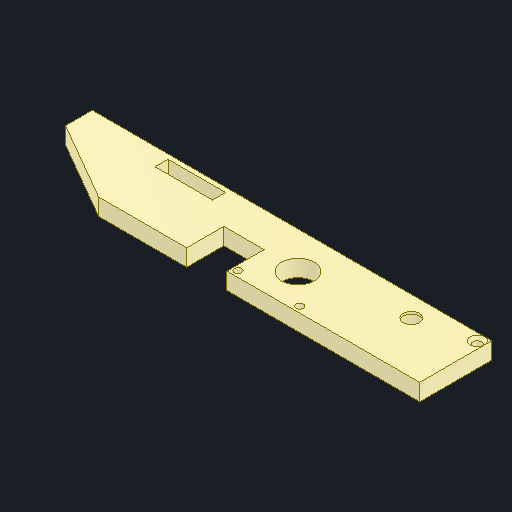
# Autodesk Inventor part: right_hold
Saved by Autodesk Inventor 2023 (Build 270158000, 158)
## iProperties
Created: 2024-04-29
Part Number: right_hold
Material: Nylon 6/6
Document SubType Name: Modeling
Designer: szymo
Density: 1.13 g/cm^3
Appearance: Nylon 6
Mass: 31.6817 g
Surface Area: 122.994 cm^2
Volume: 28.0369 cm^3
Author: szymo
Autodesk Inventor part; units mm, degrees
(part 1 of 2)
ref_plane "YZ Plane" through (0, 0, 0) normal (1, 0, 0) x (0, 1, 0)
ref_plane "XZ Plane" through (0, 0, 0) normal (0, 1, 0) x (-1, 0, 0)
ref_plane "XY Plane" through (0, 0, 0) normal (0, 0, 1) x (1, 0, 0)
sketch "Sketch1" plane through (0, 0, 0) normal (0, 0, 1) x (1, 0, 0)
  line L0 (91, -34) -> (91, 34) projected
  line L1 (91, 34) -> (41, 34) projected
  line L2 (41, 34) -> (41, 89) projected
  line L3 (41, 89) -> (-91, 89) projected
  line L4 (-91, 89) -> (-91, -89) projected
  line L5 (-91, -89) -> (41, -89) projected
  line L6 (41, -89) -> (41, -34) projected
  line L7 (41, -34) -> (91, -34) projected
  line L8 (70, 27) -> (62, 27) projected
  line L9 (91, 34) -> (-87, 34)
  line L10 (-87, 34) -> (-87, 27)
  line L11 (-87, 27) -> (91, 27)
  line L12 (91, 27) -> (91, 34)
  circle A0 centre (-83, 21.5) radius 1.2295 projected
  circle A1 centre (-83, -64.5) radius 1.2295 projected
  circle A2 centre (-83, -21.5) radius 1.2295 projected
  circle A3 centre (-83, 64.5) radius 1.2295 projected
  line L13 (-85, -72) -> (-76, -72) projected
  line L14 (-76, -72) -> (-76, -57) projected
  line L15 (-76, -57) -> (-85, -57) projected
  arc A4 (-87, -55) -> (-85, -57) centre (-85, -55) ccw projected
  line L16 (-87, -55) -> (-87, -31) projected
  arc A5 (-85, -29) -> (-87, -31) centre (-85, -31) ccw projected
  line L17 (-85, -29) -> (-76, -29) projected
  line L18 (-76, -29) -> (-76, -14) projected
  line L19 (-76, -14) -> (-85, -14) projected
  arc A6 (-87, -12) -> (-85, -14) centre (-85, -12) ccw projected
  line L20 (-87, -12) -> (-87, 12) projected
  arc A7 (-85, 14) -> (-87, 12) centre (-85, 12) ccw projected
  line L21 (-85, 14) -> (-76, 14) projected
  line L22 (-76, 14) -> (-76, 29) projected
  line L23 (-76, 29) -> (-85, 29) projected
  arc A8 (-87, 31) -> (-85, 29) centre (-85, 31) ccw projected
  line L24 (-87, 31) -> (-87, 55) projected
  arc A9 (-85, 57) -> (-87, 55) centre (-85, 55) ccw projected
  line L25 (-85, 57) -> (-76, 57) projected
  line L26 (-76, 57) -> (-76, 72) projected
  line L27 (-76, 72) -> (-85, 72) projected
  arc A10 (-87, 74) -> (-85, 72) centre (-85, 74) ccw projected
  line L28 (-87, 74) -> (-87, 89) projected
  line L29 (-91, 89) -> (-87, 89) projected
  line L30 (-91, -89) -> (-91, 89) projected
  line L31 (-91, -89) -> (-87, -89) projected
  line L32 (-87, -89) -> (-87, -74) projected
  arc A11 (-85, -72) -> (-87, -74) centre (-85, -74) ccw projected
  line L33 (-91, 89.5) -> (-86.5, 89.5)
  line L34 (-86.5, 89.5) -> (-86.5, 74)
  arc A12 (-86.5, 74) -> (-85, 72.5) centre (-85, 74) ccw
  line L35 (-85, 72.5) -> (-75.5, 72.5)
  line L36 (-75.5, 72.5) -> (-75.5, 56.5)
  line L37 (-75.5, 56.5) -> (-85, 56.5)
  arc A13 (-85, 56.5) -> (-86.5, 55) centre (-85, 55) ccw
  line L38 (-86.5, 55) -> (-86.5, 31)
  arc A14 (-86.5, 31) -> (-85, 29.5) centre (-85, 31) ccw
  line L39 (-85, 29.5) -> (-75.5, 29.5)
  line L40 (-75.5, 29.5) -> (-75.5, 13.5)
  line L41 (-75.5, 13.5) -> (-85, 13.5)
  arc A15 (-85, 13.5) -> (-86.5, 12) centre (-85, 12) ccw
  line L42 (-86.5, 12) -> (-86.5, -12)
  arc A16 (-86.5, -12) -> (-85, -13.5) centre (-85, -12) ccw
  line L43 (-85, -13.5) -> (-75.5, -13.5)
  line L44 (-75.5, -13.5) -> (-75.5, -29.5)
  line L45 (-75.5, -29.5) -> (-85, -29.5)
  arc A17 (-85, -29.5) -> (-86.5, -31) centre (-85, -31) ccw
  line L46 (-86.5, -31) -> (-86.5, -55)
  arc A18 (-86.5, -55) -> (-85, -56.5) centre (-85, -55) ccw
  line L47 (-85, -56.5) -> (-75.5, -56.5)
  line L48 (-75.5, -56.5) -> (-75.5, -72.5)
  line L49 (-75.5, -72.5) -> (-85, -72.5)
  arc A19 (-85, -72.5) -> (-86.5, -74) centre (-85, -74) ccw
  line L50 (-86.5, -74) -> (-86.5, -89.5)
  line L51 (-86.5, -89.5) -> (-91, -89.5)
  line L52 (-86.5, 31) -> (-75.5, 31)
  line L53 (-75.5, 31) -> (-75.5, 29.5)
  line L54 (-75.5, 31) -> (-75.5, 34)
  point P0 (0, 0)
  point P1 (-75.5, 27)
  point P2 (-86.5, 34)
  dimension "d6" = 0.5
  constraints: 52 end point, 16 point on circle, 8 centre point, 3 perpendicular, 2 collinear, 2 horizontal, 2 parallel, 1 point on line, 26 other
  measures "d6" distance between parallel lines of L22 L40
extrude "Extrusion1" add sketch "Sketch1" along normal blind 30 contours L11 L8 L40 L53 L54 L9 L1 L0
sketch "Sketch3" plane through (-86.5, 34, 0) normal (0, 1, 0) x (1, 0, 0)
  line L0 (-0.5, -4.5) -> (-0.5, 0) projected
  line L1 (-0.5, 0) -> (-4.5, 0) projected
  line L2 (-4.5, 0) -> (-4.5, 3.5) projected
  line L3 (-4.5, 3.5) -> (-18.5, 3.5) projected
  line L4 (-18.5, 3.5) -> (-4.5, -5.5) projected
  line L5 (-4.5, -5.5) -> (-4.5, -4.5) projected
  line L6 (-4.5, -4.5) -> (-0.5, -4.5) projected
  line L7 (-0.5, -4.5) -> (50.0525, -33.6865)
  line L8 (177.5, 0) -> (11, 0) projected
  line L9 (177.5, -30) -> (11, -30) projected
  line L10 (177.5, 0) -> (177.5, -30) projected
  line L11 (11, 0) -> (11, -30) projected
  point P0 (86.5, 0)
  point P1 (43.6673, -30)
  point P2 (11, -11.1395)
  dimension "d7" = 30
  constraints: 2 end point
  measures "d7" angle of L7 L6
extrude "Extrusion4" cut sketch "Sketch3" against normal blind 30 contours L7 L9 L11
sketch "Sketch5" plane through (-75.5, 27, 0) normal (0, -1, 0) x (1, 0, 0)
  line L0 (56.5, 7.0341) -> (57.5, 7.0341) projected
  line L1 (34.5, 7.0341) -> (56.5, 7.0341) projected
  line L2 (33.5, 7.0341) -> (33.5, 6.6226)
  line L3 (33.5, 6.6226) -> (9.5, 6.6226)
  line L4 (9.5, 6.6226) -> (9.5, 7.0341)
  line L5 (9.5, 7.0341) -> (33.5, 7.0341)
  line L6 (64.5, 7.0341) -> (64.5, 6.6226)
  line L7 (64.5, 6.6226) -> (57.5, 6.6226)
  line L8 (57.5, 6.6226) -> (57.5, 7.0341)
  line L9 (57.5, 7.0341) -> (64.5, 7.0341)
  line L10 (9.5, 2) -> (9.5, 2.6226)
  line L11 (9.5, 2.6226) -> (64.5, 2.6226)
  line L12 (64.5, 2.6226) -> (64.5, 2)
  line L13 (64.5, 2) -> (9.5, 2)
  line L14 (9.5, 7.0341) -> (64.5, 7.0341)
  line L15 (64.5, 7.0341) -> (64.5, 2)
  line L16 (64.5, 2) -> (9.5, 2)
  line L17 (9.5, 2) -> (9.5, 7.0341)
  line L18 (9.2, 7.3341) -> (64.8, 7.3341)
  line L19 (64.8, 7.3341) -> (64.8, 1.9)
  line L20 (64.8, 1.9) -> (9.2, 1.9)
  line L21 (9.2, 1.9) -> (9.2, 7.3341)
  point P0 (75.5, 0)
  dimension "d19" = 0.3
  dimension "d20" = 0.3
  dimension "d21" = 0.1
  dimension "d22" = 0.3
  constraints: 40 end point, 8 horizontal, 6 vertical, 4 parallel, 2 perpendicular, 11 other
  measures "d19" distance between parallel lines of L21 L17
  measures "d20" distance between parallel lines of L19 L15
  measures "d21" distance between parallel lines of L13 L20
  measures "d22" distance between parallel lines of L18 L1
extrude "Extrusion6" cut sketch "Sketch5" against normal blind 0.7 contours L0 L8 L7 L15 L11 L17 L3 L2 L14 L1 | L9 L6 L7 L8 | L2 L3 L4 L5 | L12 L13 L10 L11 | L18 L19 L20 L21
sketch "Sketch6" plane through (-75.5, 27, 0) normal (0, -1, 0) x (1, 0, 0)
  line L0 (33.5, 7.0341) -> (34.5, 7.0341) projected
  line L1 (34.5, 7.0341) -> (56.5, 7.0341) projected
  line L2 (56.5, 7.0341) -> (57.5, 7.0341) projected
  line L3 (64.8, 1.9) -> (9.2, 1.9) projected
  line L4 (64.8, 7.3341) -> (64.8, 1.9) projected
  line L5 (9.2, 7.3341) -> (64.8, 7.3341) projected
  line L6 (9.2, 1.9) -> (9.2, 7.3341) projected
  line L7 (33.5, 7.3341) -> (57.5, 7.3341)
  line L8 (57.5, 7.3341) -> (57.5, 1.9)
  line L9 (57.5, 1.9) -> (33.5, 1.9)
  line L10 (33.5, 1.9) -> (33.5, 7.3341)
  point P0 (75.5, 0)
  constraints: 8 end point, 4 point on line, 2 parallel, 1 horizontal, 1 perpendicular
extrude "Extrusion7" cut sketch "Sketch6" against normal up to next contours L10 L5 L8 L2 L1 L0 | L0 L1 L2 L8 L3 L10
sketch "Sketch7" plane through (0, 0, 30) normal (0, 0, 1) x (1, 0, 0)
  line L0 (10.25, -34) -> (10.25, 34) projected
  line L1 (10.25, 34) -> (-5.75, 34) projected
  line L2 (-5.75, -34) -> (-5.75, 34) projected
  line L3 (10.25, -34) -> (-5.75, -34) projected
  line L4 (-42.8327, 27) -> (91, 27) projected
  line L5 (10.25, 34) -> (-5.75, 34)
  line L6 (-5.75, 34) -> (-5.75, 27)
  line L7 (-5.75, 27) -> (10.25, 27)
  line L8 (10.25, 27) -> (10.25, 34)
  line L9 (10.65, 34) -> (-6.15, 34)
  line L10 (-6.15, 34) -> (-6.15, 27)
  line L11 (-6.15, 27) -> (10.65, 27)
  line L12 (10.65, 27) -> (10.65, 34)
  point P0 (0, 0)
  dimension "d27" = 0.4
  dimension "d28" = 0.4
  constraints: 16 end point, 4 parallel, 4 point on line, 2 horizontal, 2 perpendicular
  measures "d27" distance between parallel lines of L12 L0
  measures "d28" distance between parallel lines of L2 L10
extrude "Extrusion8" cut sketch "Sketch7" against normal blind 15.5 contours L4 L2 L1 L0 | L0 L9 L12 L4 | L4 L10 L9 L2
sketch "Sketch9" plane through (91, 27, 0) normal (0, -1, 0) x (1, 0, 0)
  arc A0 (-67.8175, 18.3693) -> (-69.7313, 19.2694) centre (-70.7618, 14.5935) ccw projected
  arc A1 (-69.7313, 19.2694) -> (-70.2869, 18.54) centre (-65.375, 15.375) ccw projected
  arc A2 (-70.2869, 18.54) -> (-68.9106, 16.9341) centre (-66.053, 20.7758) ccw projected
  arc A3 (-68.9106, 16.9341) -> (-69.111, 16.3618) centre (-65.375, 15.375) ccw projected
  arc A4 (-69.111, 16.3618) -> (-71.1884, 15.965) centre (-69.2737, 11.5765) ccw projected
  arc A5 (-71.1884, 15.965) -> (-71.2091, 15.0484) centre (-65.375, 15.375) ccw projected
  arc A6 (-71.2091, 15.0484) -> (-69.1518, 14.5581) centre (-69.098, 19.3459) ccw projected
  arc A7 (-69.1518, 14.5581) -> (-68.9775, 13.9774) centre (-65.375, 15.375) ccw projected
  arc A8 (-68.9775, 13.9774) -> (-70.425, 12.4353) centre (-66.2964, 10.0103) ccw projected
  arc A9 (-70.425, 12.4353) -> (-69.9029, 11.6815) centre (-65.375, 15.375) ccw projected
  arc A10 (-69.9029, 11.6815) -> (-67.9503, 12.4942) centre (-70.721, 16.3992) ccw projected
  arc A11 (-67.9503, 12.4942) -> (-67.468, 12.1268) centre (-65.375, 15.375) ccw projected
  arc A12 (-67.468, 12.1268) -> (-67.7326, 10.0285) centre (-62.9672, 10.4933) ccw projected
  arc A13 (-67.7326, 10.0285) -> (-66.8672, 9.7255) centre (-65.375, 15.375) ccw projected
  arc A14 (-66.8672, 9.7255) -> (-65.7652, 11.5306) centre (-70.302, 13.0613) ccw projected
  arc A15 (-65.7652, 11.5306) -> (-65.159, 11.5169) centre (-65.375, 15.375) ccw projected
  arc A16 (-65.159, 11.5169) -> (-64.1397, 9.6638) centre (-60.5576, 12.8409) ccw projected
  arc A17 (-64.1397, 9.6638) -> (-63.2615, 9.9273) centre (-65.375, 15.375) ccw projected
  arc A18 (-63.2615, 9.9273) -> (-63.431, 12.0355) centre (-68.0011, 10.6071) ccw projected
  arc A19 (-63.431, 12.0355) -> (-62.9325, 12.3807) centre (-65.375, 15.375) ccw projected
  arc A20 (-62.9325, 12.3807) -> (-61.0187, 11.4806) centre (-59.9882, 16.1565) ccw projected
  arc A21 (-61.0187, 11.4806) -> (-60.4631, 12.21) centre (-65.375, 15.375) ccw projected
  arc A22 (-60.4631, 12.21) -> (-61.8394, 13.8159) centre (-64.697, 9.9742) ccw projected
  arc A23 (-61.8394, 13.8159) -> (-61.639, 14.3882) centre (-65.375, 15.375) ccw projected
  arc A24 (-61.639, 14.3882) -> (-59.5616, 14.785) centre (-61.4763, 19.1735) ccw projected
  arc A25 (-59.5616, 14.785) -> (-59.5409, 15.7016) centre (-65.375, 15.375) ccw projected
  arc A26 (-59.5409, 15.7016) -> (-61.5982, 16.1919) centre (-61.652, 11.4041) ccw projected
  arc A27 (-61.5982, 16.1919) -> (-61.7725, 16.7726) centre (-65.375, 15.375) ccw projected
  arc A28 (-61.7725, 16.7726) -> (-60.325, 18.3147) centre (-64.4536, 20.7397) ccw projected
  arc A29 (-60.325, 18.3147) -> (-60.8471, 19.0685) centre (-65.375, 15.375) ccw projected
  arc A30 (-60.8471, 19.0685) -> (-62.7997, 18.2558) centre (-60.029, 14.3508) ccw projected
  arc A31 (-62.7997, 18.2558) -> (-63.282, 18.6232) centre (-65.375, 15.375) ccw projected
  arc A32 (-63.282, 18.6232) -> (-63.0174, 20.7215) centre (-67.7828, 20.2567) ccw projected
  arc A33 (-63.0174, 20.7215) -> (-63.8828, 21.0245) centre (-65.375, 15.375) ccw projected
  arc A34 (-63.8828, 21.0245) -> (-64.9848, 19.2194) centre (-60.448, 17.6887) ccw projected
  arc A35 (-64.9848, 19.2194) -> (-65.591, 19.2331) centre (-65.375, 15.375) ccw projected
  arc A36 (-65.591, 19.2331) -> (-66.6103, 21.0862) centre (-70.1924, 17.9091) ccw projected
  arc A37 (-66.6103, 21.0862) -> (-67.4885, 20.8227) centre (-65.375, 15.375) ccw projected
  arc A38 (-67.4885, 20.8227) -> (-67.319, 18.7145) centre (-62.7489, 20.1429) ccw projected
  arc A39 (-67.319, 18.7145) -> (-67.8175, 18.3693) centre (-65.375, 15.375) ccw projected
  circle A40 centre (-65.375, 15.375) radius 5.8433
  circle A41 centre (-65.375, 15.375) radius 6.8433
  circle A42 centre (-25, 8.5) radius 5.5 projected
  point P0 (-91, 0)
  dimension "d38" = 1
  constraints: 2 centre point, 1 coincident
  measures "d38" radial gap between concentric circles of A40 A41
extrude "Extrusion9" cut sketch "Sketch9" against normal up to next contours A39 A38 A37 A36 A35 A34 A33 A32 A31 A30 A29 A28 A27 A26 A25 A24 A23 A22 A21 A20 A19 A18 A17 A16 A15 A14 A13 A12 A11 A10 A9 A8 A7 A6 A5 A4 A3 A2 A1 A0 | A0 A40 A38 A39 | A2 A3 A4 A40 | A40 A34 A35 A36 | A6 A7 A8 A40 | A40 A30 A31 A32 | A10 A11 A12 A40 | A40 A26 A27 A28 | A14 A15 A16 A40 | A18 A19 A20 A40 | A40 A22 A23 A24 | A41
sketch "Sketch10" plane through (91, 27, 0) normal (0, -1, 0) x (1, 0, 0)
  circle A0 centre (-25, 8.5) radius 5.5 projected
  circle A1 centre (-25, 8.5) radius 5.7
  point P0 (-91, 0)
  dimension "d41" = 0.2
  constraints: 1 centre point
  measures "d41" radial gap between concentric circles of A0 A1
extrude "Extrusion10" cut sketch "Sketch10" against normal blind 6 contours A0 | A1
sketch "Sketch11" plane through (-75.5, 34, 0) normal (0, 1, 0) x (1, 0, 0)
  circle A0 centre (141.5, -8.5) radius 1.2295 projected
  line L0 (143.8461, -6.6303) -> (139.813, -6.0193) projected
  arc A1 (139.813, -6.0193) -> (139.1539, -10.3697) centre (141.5, -8.5) ccw projected
  line L1 (139.1539, -10.3697) -> (143.187, -10.9807) projected
  arc A2 (143.187, -10.9807) -> (143.8461, -6.6303) centre (141.5, -8.5) ccw projected
  circle A3 centre (141.5, -8.5) radius 5.7 projected
  circle A4 centre (141.5, -8.5) radius 3
  circle A5 centre (141.5, -8.5) radius 3.4
  point P0 (75.5, 0)
  dimension "d44" = 0.4
  constraints: 2 centre point, 1 coincident, 1 concentric
  measures "d44" radial gap between concentric circles of A4 A5
extrude "Extrusion11" cut sketch "Sketch11" against normal blind 6 contours A0 | A2 L1 A1 L0 | L0 A4 | L1 A4 | A5
sketch "Sketch12" plane through (-75.5, 27, 0) normal (0, -1, 0) x (1, 0, 0)
  circle A0 centre (111.9101, 3.5563) radius 2 projected
  point P0 (75.5, 0)
extrude "Extrusion12" cut sketch "Sketch12" against normal blind 4
sketch "Sketch13" plane through (-75.5, 34, 0) normal (0, 1, 0) x (1, 0, 0)
  circle A0 centre (114, -27.5) radius 1.55 projected
  circle A1 centre (88.25, -27.5) radius 1.55 projected
  point P0 (75.5, 0)
  constraints: 2 coincident
hole "Hole2" at (38.5, 34, 27.5) at (12.75, 34, 27.5) direction (0, -1, 0) diameter 3.1 end through all clearance for "Countersunk Flat Head Screw ISO 2009/7046" size "M2.5" standard "ISO"
sketch "Sketch14" plane through (-75.5, 34, 0) normal (0, 1, 0) x (1, 0, 0)
  circle A0 centre (114, -27.5) radius 1.55 projected
  circle A1 centre (88.25, -27.5) radius 1.55 projected
  circle A2 centre (141.5, -8.5) radius 3.4 projected
  circle A3 centre (101.125, -15.375) radius 6.8433 projected
  line L0 (69.35, -30) -> (69.35, -14.5) projected
  line L1 (69.35, -14.5) -> (86.15, -14.5) projected
  line L2 (86.15, -14.5) -> (86.15, -30) projected
  line L3 (166.5, -30) -> (86.15, -30) projected
  line L4 (166.5, 0) -> (166.5, -30) projected
  line L5 (166.5, 0) -> (0, 0) projected
  line L6 (0, 0) -> (0, -11.1395) projected
  line L7 (0, -11.1395) -> (32.6673, -30) projected
  line L8 (69.35, -30) -> (32.6673, -30) projected
  line L9 (33.5, -7.3341) -> (33.5, -1.9) projected
  line L10 (33.5, -1.9) -> (57.5, -1.9) projected
  line L11 (57.5, -1.9) -> (57.5, -7.3341) projected
  line L12 (57.5, -7.3341) -> (33.5, -7.3341) projected
  spline S0 degree 3 poles (161.425, -10.23) (161.3206, -10.2706) (161.1117, -10.3519) (160.7925, -10.4575) (160.523, -10.5345) (160.3053, -10.5877) (160.1411, -10.6234) (159.9757, -10.6537) (159.7545, -10.6901) (159.5576, -10.6964) (159.3929, -10.7314) (159.3268, -10.755) (159.2763, -10.7796) (159.2407, -10.8019) (159.2067, -10.8267) (159.1754, -10.8548) (159.1472, -10.886) (159.1224, -10.92) (159.1003, -10.9559) (159.0844, -10.9949) (159.0697, -11.0343) (159.0595, -11.0896) (159.0502, -11.1589) (159.0385, -11.228) (159.0319, -11.2837) (159.0343, -11.3258) (159.0379, -11.3677) (159.0484, -11.4085) (159.062, -11.4483) (159.0797, -11.4865) (159.1013, -11.5227) (159.1264, -11.5564) (159.1538, -11.5883) (159.1947, -11.6266) (159.2509, -11.6688) (159.3978, -11.751) (159.584, -11.8153) (159.7846, -11.9156) (159.9335, -11.9935) (160.0798, -12.0763) (160.272, -12.1917) (160.5065, -12.345) (160.7801, -12.5404) (160.9556, -12.6799) (161.0433, -12.7496) knots 0 0 0 0 0.033613 0.067227 0.100839 0.117647 0.134454 0.151261 0.168068 0.201677 0.210077 0.218473 0.222676 0.226878 0.231076 0.235279 0.239479 0.24368 0.247882 0.252083 0.256283 0.260485 0.268889 0.277292 0.281494 0.285694 0.289895 0.294097 0.298298 0.302498 0.306701 0.310899 0.315101 0.319304 0.3277 0.3361 0.369709 0.386516 0.403323 0.420131 0.436938 0.470551 0.504164 0.537777 0.537777 0.537777 0.537777 projected
  arc A4 (161.425, -10.23) -> (161.4762, -9.4749) centre (141.5, -8.5) ccw projected
  spline S1 degree 3 poles (161.438, -6.9269) (161.3417, -6.9841) (161.149, -7.0986) (160.8515, -7.2553) (160.5984, -7.3756) (160.3925, -7.464) (160.2363, -7.5263) (160.0783, -7.5834) (159.866, -7.6557) (159.6728, -7.6942) (159.5162, -7.7559) (159.4548, -7.7901) (159.4091, -7.8226) (159.3776, -7.8505) (159.3482, -7.8805) (159.3219, -7.9134) (159.2992, -7.9489) (159.2803, -7.9864) (159.2645, -8.0255) (159.2552, -8.0665) (159.2472, -8.1079) (159.2462, -8.164) (159.2485, -8.234) (159.2483, -8.304) (159.251, -8.3601) (159.2602, -8.4012) (159.2707, -8.4419) (159.2878, -8.4805) (159.3077, -8.5175) (159.3315, -8.5523) (159.3587, -8.5844) (159.3891, -8.6135) (159.4213, -8.6404) (159.468, -8.6715) (159.5304, -8.7039) (159.6888, -8.7608) (159.8831, -8.7936) (160.0974, -8.8595) (160.2571, -8.9118) (160.415, -8.9694) (160.6236, -9.0515) (160.8801, -9.1642) (161.1822, -9.3119) (161.3782, -9.4206) (161.4762, -9.4749) knots 0 0 0 0 0.033613 0.067227 0.100839 0.117647 0.134454 0.151261 0.168068 0.201677 0.210077 0.218473 0.222676 0.226878 0.231076 0.235279 0.239479 0.24368 0.247882 0.252083 0.256283 0.260485 0.268889 0.277292 0.281494 0.285694 0.289895 0.294097 0.298298 0.302498 0.306701 0.310899 0.315101 0.319304 0.3277 0.3361 0.369709 0.386516 0.403323 0.420131 0.436938 0.470551 0.504164 0.537777 0.537777 0.537777 0.537777 projected
  arc A5 (161.438, -6.9269) -> (161.3642, -6.1736) centre (141.5, -8.5) ccw projected
  spline S2 degree 3 poles (160.9072, -3.6666) (160.8216, -3.739) (160.6504, -3.8836) (160.3827, -4.0872) (160.1529, -4.2475) (159.9643, -4.3685) (159.8205, -4.4556) (159.674, -4.538) (159.4766, -4.6442) (159.2924, -4.7141) (159.148, -4.8007) (159.0931, -4.8445) (159.0533, -4.8841) (159.0269, -4.9168) (159.0028, -4.9512) (158.9823, -4.988) (158.9657, -5.0267) (158.9533, -5.0669) (158.9441, -5.108) (158.9417, -5.15) (158.9406, -5.1921) (158.9489, -5.2477) (158.9626, -5.3163) (158.974, -5.3854) (158.9859, -5.4403) (159.0017, -5.4793) (159.0188, -5.5178) (159.0419, -5.553) (159.0677, -5.5862) (159.0969, -5.6166) (159.129, -5.6438) (159.1638, -5.6675) (159.2, -5.6888) (159.2512, -5.7118) (159.318, -5.7334) (159.4837, -5.7635) (159.6807, -5.7638) (159.9029, -5.7936) (160.0691, -5.8189) (160.2343, -5.8497) (160.4535, -5.8964) (160.7251, -5.9653) (161.0474, -6.0613) (161.2586, -6.1362) (161.3642, -6.1736) knots 0 0 0 0 0.033613 0.067227 0.100839 0.117647 0.134454 0.151261 0.168068 0.201677 0.210077 0.218473 0.222676 0.226878 0.231076 0.235279 0.239479 0.24368 0.247882 0.252083 0.256283 0.260485 0.268889 0.277292 0.281494 0.285694 0.289895 0.294097 0.298298 0.302498 0.306701 0.310899 0.315101 0.319304 0.3277 0.3361 0.369709 0.386516 0.403323 0.420131 0.436938 0.470551 0.504164 0.537777 0.537777 0.537777 0.537777 projected
  arc A6 (160.9072, -3.6666) -> (160.7104, -2.9358) centre (141.5, -8.5) ccw projected
  spline S3 degree 3 poles (159.8469, -0.5383) (159.7744, -0.6237) (159.6294, -0.7945) (159.3989, -1.0394) (159.1985, -1.2353) (159.0324, -1.3857) (158.905, -1.4953) (158.774, -1.6007) (158.5968, -1.738) (158.4265, -1.8372) (158.2984, -1.9464) (158.2514, -1.9986) (158.2188, -2.0442) (158.1981, -2.0808) (158.1799, -2.1188) (158.1658, -2.1584) (158.1558, -2.1993) (158.1502, -2.241) (158.1479, -2.2831) (158.1524, -2.3249) (158.1583, -2.3666) (158.1756, -2.4201) (158.2005, -2.4855) (158.223, -2.5517) (158.2438, -2.6039) (158.2658, -2.6398) (158.289, -2.6749) (158.3176, -2.7059) (158.3485, -2.7344) (158.3823, -2.7595) (158.4185, -2.7811) (158.4566, -2.7987) (158.4959, -2.8138) (158.5502, -2.828) (158.6196, -2.8384) (158.788, -2.8408) (158.9824, -2.8087) (159.2065, -2.8015) (159.3745, -2.7991) (159.5426, -2.8023) (159.7665, -2.8123) (160.0457, -2.8355) (160.3794, -2.8771) (160.6001, -2.9163) (160.7104, -2.9358) knots 0 0 0 0 0.033613 0.067227 0.100839 0.117647 0.134454 0.151261 0.168068 0.201677 0.210077 0.218473 0.222676 0.226878 0.231076 0.235279 0.239479 0.24368 0.247882 0.252083 0.256283 0.260485 0.268889 0.277292 0.281494 0.285694 0.289895 0.294097 0.298298 0.302498 0.306701 0.310899 0.315101 0.319304 0.3277 0.3361 0.369709 0.386516 0.403323 0.420131 0.436938 0.470551 0.504164 0.537777 0.537777 0.537777 0.537777 projected
  arc A7 (159.8469, -0.5383) -> (159.5326, 0.1502) centre (141.5, -8.5) ccw projected
  spline S4 degree 3 poles (158.2863, 2.373) (158.2288, 2.2768) (158.1138, 2.0844) (157.9268, 1.8049) (157.7614, 1.5787) (157.6223, 1.403) (157.5147, 1.2739) (157.4028, 1.1484) (157.2506, 0.9839) (157.099, 0.8579) (156.9906, 0.7292) (156.9529, 0.6699) (156.9282, 0.6196) (156.9138, 0.58) (156.9021, 0.5396) (156.8947, 0.4982) (156.8916, 0.4562) (156.8929, 0.4142) (156.8976, 0.3723) (156.9089, 0.3318) (156.9216, 0.2916) (156.9475, 0.2417) (156.9827, 0.1813) (157.0159, 0.1197) (157.045, 0.0716) (157.0726, 0.0398) (157.1013, 0.009) (157.1346, -0.0168) (157.1698, -0.0399) (157.2072, -0.0591) (157.2464, -0.0744) (157.287, -0.0855) (157.3282, -0.0939) (157.384, -0.099) (157.4543, -0.0978) (157.6207, -0.0725) (157.8072, -0.0088) (158.027, 0.0352) (158.1924, 0.0652) (158.3587, 0.0897) (158.5812, 0.1167) (158.8604, 0.1398) (159.1964, 0.1536) (159.4205, 0.1513) (159.5326, 0.1502) knots 0 0 0 0 0.033613 0.067227 0.100839 0.117647 0.134454 0.151261 0.168068 0.201677 0.210077 0.218473 0.222676 0.226878 0.231076 0.235279 0.239479 0.24368 0.247882 0.252083 0.256283 0.260485 0.268889 0.277292 0.281494 0.285694 0.289895 0.294097 0.298298 0.302498 0.306701 0.310899 0.315101 0.319304 0.3277 0.3361 0.369709 0.386516 0.403323 0.420131 0.436938 0.470551 0.504164 0.537777 0.537777 0.537777 0.537777 projected
  arc A8 (158.2863, 2.373) -> (157.8629, 3.0003) centre (141.5, -8.5) ccw projected
  spline S5 degree 3 poles (156.2677, 4.9876) (156.2268, 4.8833) (156.1451, 4.6746) (156.0066, 4.3682) (155.8807, 4.1178) (155.7725, 3.9216) (155.6875, 3.7765) (155.5978, 3.6344) (155.4748, 3.447) (155.346, 3.2978) (155.2603, 3.153) (155.2328, 3.0883) (155.2167, 3.0346) (155.209, 2.9932) (155.2042, 2.9514) (155.2037, 2.9094) (155.2075, 2.8674) (155.2158, 2.8262) (155.2272, 2.7856) (155.2451, 2.7475) (155.2642, 2.71) (155.2979, 2.6651) (155.3427, 2.6113) (155.3856, 2.5559) (155.4221, 2.5133) (155.4546, 2.4865) (155.4879, 2.4608) (155.5251, 2.4408) (155.5636, 2.4239) (155.6037, 2.4111) (155.6448, 2.4025) (155.6867, 2.3982) (155.7287, 2.3967) (155.7847, 2.4008) (155.8537, 2.4136) (156.0137, 2.466) (156.1872, 2.5594) (156.3968, 2.6391) (156.5549, 2.6959) (156.7149, 2.7474) (156.9299, 2.8107) (157.2016, 2.8794) (157.5307, 2.9483) (157.7521, 2.983) (157.8629, 3.0003) knots 0 0 0 0 0.033613 0.067227 0.100839 0.117647 0.134454 0.151261 0.168068 0.201677 0.210077 0.218473 0.222676 0.226878 0.231076 0.235279 0.239479 0.24368 0.247882 0.252083 0.256283 0.260485 0.268889 0.277292 0.281494 0.285694 0.289895 0.294097 0.298298 0.302498 0.306701 0.310899 0.315101 0.319304 0.3277 0.3361 0.369709 0.386516 0.403323 0.420131 0.436938 0.470551 0.504164 0.537777 0.537777 0.537777 0.537777 projected
  arc A9 (156.2677, 4.9876) -> (155.7468, 5.5367) centre (141.5, -8.5) ccw projected
  spline S6 degree 3 poles (153.8463, 7.2343) (153.8232, 7.1247) (153.7769, 6.9054) (153.6907, 6.5804) (153.6078, 6.3127) (153.5333, 6.1013) (153.4734, 5.9443) (153.4083, 5.7893) (153.3178, 5.5842) (153.2153, 5.4159) (153.1546, 5.2589) (153.1382, 5.1906) (153.1311, 5.135) (153.1303, 5.0929) (153.1325, 5.0509) (153.1389, 5.0093) (153.1496, 4.9686) (153.1645, 4.9293) (153.1825, 4.8911) (153.2064, 4.8565) (153.2314, 4.8226) (153.272, 4.7839) (153.325, 4.7381) (153.3764, 4.6906) (153.4195, 4.6546) (153.456, 4.6335) (153.4931, 4.6137) (153.533, 4.6001) (153.5737, 4.5897) (153.6154, 4.5837) (153.6574, 4.5819) (153.6994, 4.5846) (153.7411, 4.5901) (153.7956, 4.6033) (153.8616, 4.6273) (154.0108, 4.7053) (154.1665, 4.826) (154.3602, 4.9391) (154.5068, 5.0211) (154.6562, 5.0983) (154.8578, 5.1961) (155.1145, 5.3086) (155.4277, 5.4308) (155.6405, 5.5014) (155.7468, 5.5367) knots 0 0 0 0 0.033613 0.067227 0.100839 0.117647 0.134454 0.151261 0.168068 0.201677 0.210077 0.218473 0.222676 0.226878 0.231076 0.235279 0.239479 0.24368 0.247882 0.252083 0.256283 0.260485 0.268889 0.277292 0.281494 0.285694 0.289895 0.294097 0.298298 0.302498 0.306701 0.310899 0.315101 0.319304 0.3277 0.3361 0.369709 0.386516 0.403323 0.420131 0.436938 0.470551 0.504164 0.537777 0.537777 0.537777 0.537777 projected
  arc A10 (153.8463, 7.2343) -> (153.2421, 7.6902) centre (141.5, -8.5) ccw projected
  spline S7 degree 3 poles (151.0881, 9.0519) (151.0833, 8.9399) (151.0738, 8.716) (151.0423, 8.3812) (151.0046, 8.1035) (150.9659, 7.8828) (150.9326, 7.718) (150.894, 7.5544) (150.8384, 7.3372) (150.765, 7.1544) (150.731, 6.9895) (150.726, 6.9194) (150.7282, 6.8634) (150.7344, 6.8218) (150.7434, 6.7807) (150.7566, 6.7408) (150.7738, 6.7023) (150.795, 6.666) (150.819, 6.6314) (150.8483, 6.6012) (150.8785, 6.5719) (150.925, 6.5403) (150.9848, 6.5039) (151.0433, 6.4655) (151.0918, 6.4371) (151.1312, 6.4223) (151.1711, 6.4088) (151.2127, 6.402) (151.2546, 6.3984) (151.2967, 6.3994) (151.3384, 6.4046) (151.3794, 6.4141) (151.4196, 6.4263) (151.4712, 6.4484) (151.5324, 6.4829) (151.6667, 6.5844) (151.8004, 6.7291) (151.9728, 6.8725) (152.1039, 6.9776) (152.2385, 7.0783) (152.4213, 7.2079) (152.656, 7.3611) (152.9449, 7.5332) (153.143, 7.6379) (153.2421, 7.6902) knots 0 0 0 0 0.033613 0.067227 0.100839 0.117647 0.134454 0.151261 0.168068 0.201677 0.210077 0.218473 0.222676 0.226878 0.231076 0.235279 0.239479 0.24368 0.247882 0.252083 0.256283 0.260485 0.268889 0.277292 0.281494 0.285694 0.289895 0.294097 0.298298 0.302498 0.306701 0.310899 0.315101 0.319304 0.3277 0.3361 0.369709 0.386516 0.403323 0.420131 0.436938 0.470551 0.504164 0.537777 0.537777 0.537777 0.537777 projected
  arc A11 (151.0881, 9.0519) -> (150.4172, 9.4021) centre (141.5, -8.5) ccw projected
  spline S8 degree 3 poles (148.0684, 10.3906) (148.0821, 10.2794) (148.1096, 10.057) (148.1336, 9.7216) (148.1421, 9.4415) (148.1403, 9.2174) (148.1346, 9.0494) (148.1234, 8.8817) (148.1043, 8.6583) (148.0621, 8.4659) (148.0556, 8.2976) (148.0622, 8.2277) (148.0736, 8.1728) (148.0866, 8.1328) (148.1022, 8.0937) (148.1218, 8.0565) (148.1451, 8.0214) (148.172, 7.9891) (148.2014, 7.9589) (148.2352, 7.9339) (148.2699, 7.91) (148.3209, 7.8865) (148.3859, 7.8604) (148.4499, 7.8322) (148.5024, 7.8121) (148.5437, 7.804) (148.5853, 7.7973) (148.6274, 7.7974) (148.6693, 7.8008) (148.7107, 7.8086) (148.751, 7.8206) (148.7899, 7.8368) (148.8275, 7.8555) (148.8748, 7.8857) (148.9294, 7.9298) (149.0452, 8.0521) (149.1533, 8.2168) (149.2997, 8.3866) (149.4118, 8.5118) (149.528, 8.6333) (149.6869, 8.7913) (149.8932, 8.981) (150.1498, 9.1983) (150.328, 9.3341) (150.4172, 9.4021) knots 0 0 0 0 0.033613 0.067227 0.100839 0.117647 0.134454 0.151261 0.168068 0.201677 0.210077 0.218473 0.222676 0.226878 0.231076 0.235279 0.239479 0.24368 0.247882 0.252083 0.256283 0.260485 0.268889 0.277292 0.281494 0.285694 0.289895 0.294097 0.298298 0.302498 0.306701 0.310899 0.315101 0.319304 0.3277 0.3361 0.369709 0.386516 0.403323 0.420131 0.436938 0.470551 0.504164 0.537777 0.537777 0.537777 0.537777 projected
  arc A12 (148.0684, 10.3906) -> (147.349, 10.6256) centre (141.5, -8.5) ccw projected
  spline S9 degree 3 poles (144.8695, 11.2141) (144.9014, 11.1067) (144.9651, 10.8918) (145.044, 10.5649) (145.0984, 10.29) (145.1335, 10.0687) (145.1555, 9.902) (145.1721, 9.7348) (145.1901, 9.5113) (145.1801, 9.3145) (145.2014, 9.1475) (145.2194, 9.0797) (145.2397, 9.0274) (145.2591, 8.99) (145.2809, 8.9541) (145.3064, 8.9206) (145.3352, 8.8898) (145.367, 8.8623) (145.4009, 8.8374) (145.4384, 8.8183) (145.4766, 8.8004) (145.5308, 8.7857) (145.5991, 8.7707) (145.667, 8.7534) (145.722, 8.7422) (145.7641, 8.741) (145.8062, 8.7412) (145.8477, 8.7482) (145.8885, 8.7585) (145.928, 8.773) (145.9658, 8.7915) (146.0015, 8.8138) (146.0356, 8.8385) (146.0772, 8.8761) (146.1238, 8.9286) (146.2179, 9.0682) (146.2974, 9.2485) (146.4139, 9.4401) (146.5038, 9.582) (146.5984, 9.721) (146.7292, 9.903) (146.9014, 10.1241) (147.1188, 10.3806) (147.2722, 10.544) (147.349, 10.6256) knots 0 0 0 0 0.033613 0.067227 0.100839 0.117647 0.134454 0.151261 0.168068 0.201677 0.210077 0.218473 0.222676 0.226878 0.231076 0.235279 0.239479 0.24368 0.247882 0.252083 0.256283 0.260485 0.268889 0.277292 0.281494 0.285694 0.289895 0.294097 0.298298 0.302498 0.306701 0.310899 0.315101 0.319304 0.3277 0.3361 0.369709 0.386516 0.403323 0.420131 0.436938 0.470551 0.504164 0.537777 0.537777 0.537777 0.537777 projected
  arc A13 (144.8695, 11.2141) -> (144.1212, 11.3275) centre (141.5, -8.5) ccw projected
  spline S10 degree 3 poles (141.5787, 11.4998) (141.6278, 11.3991) (141.726, 11.1976) (141.8576, 10.8882) (141.9566, 10.6261) (142.0276, 10.4135) (142.0768, 10.2527) (142.1207, 10.0905) (142.1752, 9.873) (142.1977, 9.6773) (142.2462, 9.5161) (142.2752, 9.4521) (142.3038, 9.4039) (142.3291, 9.3702) (142.3565, 9.3384) (142.3871, 9.3095) (142.4206, 9.2839) (142.4565, 9.262) (142.4941, 9.243) (142.5342, 9.2304) (142.5748, 9.219) (142.6307, 9.2134) (142.7006, 9.2098) (142.7703, 9.2039) (142.8265, 9.2019) (142.8682, 9.2077) (142.9096, 9.2148) (142.9495, 9.2286) (142.988, 9.2455) (143.0246, 9.2663) (143.0588, 9.2907) (143.0903, 9.3186) (143.1199, 9.3485) (143.1547, 9.3925) (143.1921, 9.452) (143.2619, 9.6052) (143.3107, 9.7961) (143.394, 10.0042) (143.4594, 10.159) (143.5298, 10.3117) (143.6289, 10.5127) (143.7623, 10.7591) (143.9345, 11.0479) (144.059, 11.2343) (144.1212, 11.3275) knots 0 0 0 0 0.033613 0.067227 0.100839 0.117647 0.134454 0.151261 0.168068 0.201677 0.210077 0.218473 0.222676 0.226878 0.231076 0.235279 0.239479 0.24368 0.247882 0.252083 0.256283 0.260485 0.268889 0.277292 0.281494 0.285694 0.289895 0.294097 0.298298 0.302498 0.306701 0.310899 0.315101 0.319304 0.3277 0.3361 0.369709 0.386516 0.403323 0.420131 0.436938 0.470551 0.504164 0.537777 0.537777 0.537777 0.537777 projected
  arc A14 (141.5787, 11.4998) -> (140.822, 11.4885) centre (141.5, -8.5) ccw projected
  spline S11 degree 3 poles (138.2858, 11.24) (138.3508, 11.1488) (138.4808, 10.9662) (138.6616, 10.6826) (138.8023, 10.4404) (138.9074, 10.2424) (138.9823, 10.0919) (139.0523, 9.9391) (139.1419, 9.7336) (139.1963, 9.5442) (139.2707, 9.3932) (139.3098, 9.3348) (139.346, 9.292) (139.3764, 9.2629) (139.4087, 9.236) (139.4437, 9.2126) (139.4809, 9.1929) (139.5199, 9.1772) (139.5601, 9.1646) (139.6018, 9.1588) (139.6437, 9.1542) (139.6997, 9.1579) (139.7693, 9.1659) (139.839, 9.1715) (139.8947, 9.1788) (139.9349, 9.1914) (139.9746, 9.2052) (140.0117, 9.2254) (140.0469, 9.2483) (140.0796, 9.2749) (140.1093, 9.3047) (140.1358, 9.3373) (140.16, 9.3717) (140.1872, 9.4208) (140.2142, 9.4856) (140.2579, 9.6482) (140.2745, 9.8446) (140.3225, 10.0636) (140.3615, 10.227) (140.4058, 10.3892) (140.4704, 10.6038) (140.5615, 10.8688) (140.6838, 11.182) (140.7759, 11.3863) (140.822, 11.4885) knots 0 0 0 0 0.033613 0.067227 0.100839 0.117647 0.134454 0.151261 0.168068 0.201677 0.210077 0.218473 0.222676 0.226878 0.231076 0.235279 0.239479 0.24368 0.247882 0.252083 0.256283 0.260485 0.268889 0.277292 0.281494 0.285694 0.289895 0.294097 0.298298 0.302498 0.306701 0.310899 0.315101 0.319304 0.3277 0.3361 0.369709 0.386516 0.403323 0.420131 0.436938 0.470551 0.504164 0.537777 0.537777 0.537777 0.537777 projected
  arc A15 (138.2858, 11.24) -> (137.5412, 11.1043) centre (141.5, -8.5) ccw projected
  spline S12 degree 3 poles (135.0805, 10.4418) (135.1597, 10.3624) (135.3179, 10.2038) (135.5429, 9.9538) (135.7216, 9.738) (135.8579, 9.56) (135.9566, 9.424) (136.0507, 9.2847) (136.1729, 9.0968) (136.2577, 8.9189) (136.356, 8.7822) (136.4042, 8.7311) (136.4469, 8.6948) (136.4817, 8.6711) (136.518, 8.6499) (136.5563, 8.6326) (136.5963, 8.6192) (136.6373, 8.6102) (136.6791, 8.6044) (136.7212, 8.6055) (136.7632, 8.6079) (136.8179, 8.6207) (136.8852, 8.6401) (136.953, 8.6571) (137.0068, 8.6735) (137.0443, 8.6925) (137.0813, 8.7127) (137.1145, 8.7387) (137.1454, 8.7671) (137.1733, 8.7987) (137.1977, 8.8329) (137.2185, 8.8695) (137.2367, 8.9074) (137.2554, 8.9603) (137.2714, 9.0287) (137.2877, 9.1963) (137.2718, 9.3927) (137.2831, 9.6166) (137.2946, 9.7842) (137.3117, 9.9515) (137.3401, 10.1738) (137.3863, 10.4501) (137.4554, 10.7792) (137.5126, 10.9959) (137.5412, 11.1043) knots 0 0 0 0 0.033613 0.067227 0.100839 0.117647 0.134454 0.151261 0.168068 0.201677 0.210077 0.218473 0.222676 0.226878 0.231076 0.235279 0.239479 0.24368 0.247882 0.252083 0.256283 0.260485 0.268889 0.277292 0.281494 0.285694 0.289895 0.294097 0.298298 0.302498 0.306701 0.310899 0.315101 0.319304 0.3277 0.3361 0.369709 0.386516 0.403323 0.420131 0.436938 0.470551 0.504164 0.537777 0.537777 0.537777 0.537777 projected
  arc A16 (135.0805, 10.4418) -> (134.3685, 10.1853) centre (141.5, -8.5) ccw projected
  spline S13 degree 3 poles (132.0504, 9.1268) (132.1415, 9.0616) (132.3237, 8.9311) (132.5868, 8.7216) (132.7986, 8.5382) (132.9622, 8.3851) (133.082, 8.2671) (133.1978, 8.1453) (133.3492, 7.98) (133.4622, 7.8185) (133.5816, 7.6998) (133.6375, 7.6574) (133.6856, 7.6286) (133.7239, 7.611) (133.7632, 7.596) (133.8038, 7.5852) (133.8454, 7.5786) (133.8874, 7.5765) (133.9295, 7.5776) (133.9709, 7.5856) (134.0119, 7.5949) (134.0638, 7.6166) (134.1269, 7.6467) (134.1911, 7.6747) (134.2414, 7.6997) (134.2753, 7.7247) (134.3084, 7.7506) (134.3369, 7.7817) (134.3628, 7.8149) (134.385, 7.8506) (134.4035, 7.8884) (134.4179, 7.9279) (134.4297, 7.9683) (134.4394, 8.0235) (134.444, 8.0936) (134.4325, 8.2616) (134.3845, 8.4527) (134.3587, 8.6754) (134.3425, 8.8427) (134.3318, 9.0104) (134.3232, 9.2344) (134.3233, 9.5146) (134.3373, 9.8506) (134.3581, 10.0737) (134.3685, 10.1853) knots 0 0 0 0 0.033613 0.067227 0.100839 0.117647 0.134454 0.151261 0.168068 0.201677 0.210077 0.218473 0.222676 0.226878 0.231076 0.235279 0.239479 0.24368 0.247882 0.252083 0.256283 0.260485 0.268889 0.277292 0.281494 0.285694 0.289895 0.294097 0.298298 0.302498 0.306701 0.310899 0.315101 0.319304 0.3277 0.3361 0.369709 0.386516 0.403323 0.420131 0.436938 0.470551 0.504164 0.537777 0.537777 0.537777 0.537777 projected
  arc A17 (132.0504, 9.1268) -> (131.3902, 8.7567) centre (141.5, -8.5) ccw projected
  spline S14 degree 3 poles (129.278, 7.331) (129.3786, 7.2817) (129.5798, 7.183) (129.8737, 7.0197) (130.1129, 6.8736) (130.2995, 6.7495) (130.437, 6.6528) (130.5713, 6.5517) (130.7479, 6.4136) (130.8859, 6.273) (131.0232, 6.1755) (131.0853, 6.1429) (131.1375, 6.1224) (131.1781, 6.1113) (131.2194, 6.103) (131.2613, 6.0991) (131.3034, 6.0994) (131.3451, 6.1042) (131.3865, 6.1123) (131.4259, 6.127) (131.4649, 6.1429) (131.5125, 6.1728) (131.5698, 6.2129) (131.6285, 6.2511) (131.674, 6.284) (131.7034, 6.3142) (131.7317, 6.3453) (131.7547, 6.3807) (131.7748, 6.4176) (131.7908, 6.4565) (131.8028, 6.4969) (131.8106, 6.5382) (131.8155, 6.58) (131.816, 6.636) (131.809, 6.7059) (131.77, 6.8697) (131.6912, 7.0503) (131.6291, 7.2657) (131.5856, 7.4281) (131.5474, 7.5918) (131.5021, 7.8113) (131.4561, 8.0877) (131.4146, 8.4214) (131.3983, 8.6449) (131.3902, 8.7567) knots 0 0 0 0 0.033613 0.067227 0.100839 0.117647 0.134454 0.151261 0.168068 0.201677 0.210077 0.218473 0.222676 0.226878 0.231076 0.235279 0.239479 0.24368 0.247882 0.252083 0.256283 0.260485 0.268889 0.277292 0.281494 0.285694 0.289895 0.294097 0.298298 0.302498 0.306701 0.310899 0.315101 0.319304 0.3277 0.3361 0.369709 0.386516 0.403323 0.420131 0.436938 0.470551 0.504164 0.537777 0.537777 0.537777 0.537777 projected
  arc A18 (129.278, 7.331) -> (128.6877, 6.8573) centre (141.5, -8.5) ccw projected
  spline S15 degree 3 poles (126.839, 5.1034) (126.9463, 5.0713) (127.161, 5.0071) (127.4779, 4.8944) (127.7378, 4.7897) (127.9422, 4.698) (128.0938, 4.6253) (128.2429, 4.5476) (128.4398, 4.4405) (128.5991, 4.3245) (128.7505, 4.251) (128.8172, 4.229) (128.8721, 4.2173) (128.914, 4.2131) (128.956, 4.2117) (128.998, 4.2147) (129.0394, 4.222) (129.0799, 4.2336) (129.1193, 4.2484) (129.1558, 4.2694) (129.1916, 4.2915) (129.2336, 4.3288) (129.2836, 4.3778) (129.3352, 4.4251) (129.3746, 4.4651) (129.3986, 4.4997) (129.4215, 4.535) (129.4383, 4.5737) (129.452, 4.6134) (129.4615, 4.6545) (129.4667, 4.6962) (129.4675, 4.7383) (129.4655, 4.7803) (129.4568, 4.8357) (129.4384, 4.9035) (129.3729, 5.0586) (129.2655, 5.2237) (129.1688, 5.426) (129.0992, 5.579) (129.0345, 5.7342) (128.9538, 5.9432) (128.8629, 6.2083) (128.767, 6.5306) (128.7142, 6.7484) (128.6877, 6.8573) knots 0 0 0 0 0.033613 0.067227 0.100839 0.117647 0.134454 0.151261 0.168068 0.201677 0.210077 0.218473 0.222676 0.226878 0.231076 0.235279 0.239479 0.24368 0.247882 0.252083 0.256283 0.260485 0.268889 0.277292 0.281494 0.285694 0.289895 0.294097 0.298298 0.302498 0.306701 0.310899 0.315101 0.319304 0.3277 0.3361 0.369709 0.386516 0.403323 0.420131 0.436938 0.470551 0.504164 0.537777 0.537777 0.537777 0.537777 projected
  arc A19 (126.839, 5.1034) -> (126.3348, 4.539) centre (141.5, -8.5) ccw projected
  spline S16 degree 3 poles (124.7999, 2.5048) (124.911, 2.4908) (125.1334, 2.4628) (125.4645, 2.4037) (125.738, 2.3432) (125.9548, 2.2864) (126.1163, 2.2397) (126.2761, 2.1876) (126.488, 2.1143) (126.6642, 2.0261) (126.8257, 1.9786) (126.8951, 1.9678) (126.9511, 1.9654) (126.9931, 1.9681) (127.0348, 1.9737) (127.0757, 1.9836) (127.1154, 1.9976) (127.1534, 2.0156) (127.1899, 2.0367) (127.2224, 2.0634) (127.2541, 2.0911) (127.2894, 2.1349) (127.3306, 2.1914) (127.3737, 2.2466) (127.406, 2.2925) (127.424, 2.3306) (127.4407, 2.3692) (127.451, 2.4101) (127.458, 2.4516) (127.4605, 2.4936) (127.4588, 2.5356) (127.4527, 2.5772) (127.4438, 2.6183) (127.4261, 2.6716) (127.3967, 2.7354) (127.3067, 2.8776) (127.1735, 3.0228) (127.0449, 3.2064) (126.951, 3.3458) (126.8617, 3.4883) (126.7476, 3.6812) (126.6143, 3.9277) (126.4667, 4.2298) (126.3787, 4.4359) (126.3348, 4.539) knots 0 0 0 0 0.033613 0.067227 0.100839 0.117647 0.134454 0.151261 0.168068 0.201677 0.210077 0.218473 0.222676 0.226878 0.231076 0.235279 0.239479 0.24368 0.247882 0.252083 0.256283 0.260485 0.268889 0.277292 0.281494 0.285694 0.289895 0.294097 0.298298 0.302498 0.306701 0.310899 0.315101 0.319304 0.3277 0.3361 0.369709 0.386516 0.403323 0.420131 0.436938 0.470551 0.504164 0.537777 0.537777 0.537777 0.537777 projected
  arc A20 (124.7999, 2.5048) -> (124.3954, 1.8651) centre (141.5, -8.5) ccw projected
  spline S17 degree 3 poles (123.2163, -0.3941) (123.3283, -0.3896) (123.5522, -0.3806) (123.8885, -0.3843) (124.1683, -0.399) (124.3915, -0.4193) (124.5584, -0.4389) (124.7246, -0.4639) (124.9457, -0.5013) (125.134, -0.5593) (125.3011, -0.5797) (125.3713, -0.5788) (125.427, -0.572) (125.468, -0.5624) (125.5082, -0.55) (125.5469, -0.5336) (125.5838, -0.5132) (125.6182, -0.4892) (125.6508, -0.4624) (125.6785, -0.4307) (125.7051, -0.3981) (125.7327, -0.3492) (125.7641, -0.2866) (125.7975, -0.2251) (125.8219, -0.1745) (125.8333, -0.134) (125.8435, -0.0931) (125.8469, -0.0511) (125.8469, -0.0091) (125.8425, 0.0328) (125.8339, 0.074) (125.821, 0.114) (125.8055, 0.1531) (125.7793, 0.2027) (125.7398, 0.2608) (125.6275, 0.3863) (125.4723, 0.5076) (125.3152, 0.6675) (125.1996, 0.7896) (125.0881, 0.9154) (124.9438, 1.0869) (124.7718, 1.3081) (124.5765, 1.5818) (124.4558, 1.7706) (124.3954, 1.8651) knots 0 0 0 0 0.033613 0.067227 0.100839 0.117647 0.134454 0.151261 0.168068 0.201677 0.210077 0.218473 0.222676 0.226878 0.231076 0.235279 0.239479 0.24368 0.247882 0.252083 0.256283 0.260485 0.268889 0.277292 0.281494 0.285694 0.289895 0.294097 0.298298 0.302498 0.306701 0.310899 0.315101 0.319304 0.3277 0.3361 0.369709 0.386516 0.403323 0.420131 0.436938 0.470551 0.504164 0.537777 0.537777 0.537777 0.537777 projected
  arc A21 (123.2163, -0.3941) -> (122.9227, -1.0916) centre (141.5, -8.5) ccw projected
  spline S18 degree 3 poles (122.1315, -3.514) (122.2412, -3.4911) (122.4606, -3.4454) (122.7929, -3.3938) (123.0713, -3.3622) (123.2948, -3.3455) (123.4627, -3.3373) (123.6307, -3.3346) (123.8549, -3.3352) (124.0502, -3.3614) (124.2184, -3.3539) (124.2875, -3.3415) (124.3413, -3.3256) (124.3801, -3.3094) (124.4178, -3.2906) (124.4533, -3.268) (124.4863, -3.2419) (124.5163, -3.2125) (124.544, -3.1807) (124.5661, -3.1449) (124.587, -3.1084) (124.6062, -3.0556) (124.6268, -2.9887) (124.6497, -2.9225) (124.6654, -2.8686) (124.67, -2.8267) (124.6733, -2.7848) (124.6697, -2.7428) (124.6628, -2.7013) (124.6516, -2.6607) (124.6363, -2.6215) (124.617, -2.5841) (124.5953, -2.5481) (124.5612, -2.5035) (124.5128, -2.4527) (124.3814, -2.3474) (124.2083, -2.2533) (124.027, -2.1214) (123.8929, -2.0201) (123.7622, -1.9143) (123.5917, -1.7689) (123.3856, -1.5791) (123.1479, -1.3413) (122.9978, -1.1748) (122.9227, -1.0916) knots 0 0 0 0 0.033613 0.067227 0.100839 0.117647 0.134454 0.151261 0.168068 0.201677 0.210077 0.218473 0.222676 0.226878 0.231076 0.235279 0.239479 0.24368 0.247882 0.252083 0.256283 0.260485 0.268889 0.277292 0.281494 0.285694 0.289895 0.294097 0.298298 0.302498 0.306701 0.310899 0.315101 0.319304 0.3277 0.3361 0.369709 0.386516 0.403323 0.420131 0.436938 0.470551 0.504164 0.537777 0.537777 0.537777 0.537777 projected
  arc A22 (122.1315, -3.514) -> (121.9567, -4.2504) centre (141.5, -8.5) ccw projected
  spline S19 degree 3 poles (121.575, -6.77) (121.6794, -6.7294) (121.8883, -6.6481) (122.2075, -6.5425) (122.477, -6.4655) (122.6947, -6.4123) (122.8589, -6.3766) (123.0243, -6.3463) (123.2455, -6.3099) (123.4424, -6.3036) (123.6071, -6.2686) (123.6732, -6.245) (123.7237, -6.2204) (123.7593, -6.1981) (123.7933, -6.1733) (123.8246, -6.1452) (123.8528, -6.114) (123.8776, -6.08) (123.8997, -6.0441) (123.9156, -6.0051) (123.9303, -5.9657) (123.9405, -5.9104) (123.9498, -5.8411) (123.9615, -5.772) (123.9681, -5.7163) (123.9657, -5.6742) (123.9621, -5.6323) (123.9516, -5.5915) (123.938, -5.5517) (123.9203, -5.5135) (123.8987, -5.4773) (123.8736, -5.4436) (123.8462, -5.4117) (123.8053, -5.3734) (123.7491, -5.3312) (123.6022, -5.249) (123.416, -5.1847) (123.2154, -5.0844) (123.0665, -5.0065) (122.9202, -4.9237) (122.728, -4.8083) (122.4935, -4.655) (122.2199, -4.4596) (122.0444, -4.3201) (121.9567, -4.2504) knots 0 0 0 0 0.033613 0.067227 0.100839 0.117647 0.134454 0.151261 0.168068 0.201677 0.210077 0.218473 0.222676 0.226878 0.231076 0.235279 0.239479 0.24368 0.247882 0.252083 0.256283 0.260485 0.268889 0.277292 0.281494 0.285694 0.289895 0.294097 0.298298 0.302498 0.306701 0.310899 0.315101 0.319304 0.3277 0.3361 0.369709 0.386516 0.403323 0.420131 0.436938 0.470551 0.504164 0.537777 0.537777 0.537777 0.537777 projected
  arc A23 (121.575, -6.77) -> (121.5238, -7.5251) centre (141.5, -8.5) ccw projected
  spline S20 degree 3 poles (121.562, -10.0731) (121.6583, -10.0159) (121.851, -9.9014) (122.1485, -9.7447) (122.4016, -9.6244) (122.6075, -9.536) (122.7637, -9.4737) (122.9217, -9.4166) (123.134, -9.3443) (123.3272, -9.3058) (123.4838, -9.2441) (123.5452, -9.2099) (123.5909, -9.1774) (123.6224, -9.1495) (123.6518, -9.1195) (123.6781, -9.0866) (123.7008, -9.0511) (123.7197, -9.0136) (123.7355, -8.9745) (123.7448, -8.9335) (123.7528, -8.8921) (123.7538, -8.836) (123.7515, -8.766) (123.7517, -8.696) (123.749, -8.6399) (123.7398, -8.5988) (123.7293, -8.5581) (123.7122, -8.5195) (123.6923, -8.4825) (123.6685, -8.4477) (123.6413, -8.4156) (123.6109, -8.3865) (123.5787, -8.3596) (123.532, -8.3285) (123.4696, -8.2961) (123.3112, -8.2392) (123.1169, -8.2064) (122.9026, -8.1405) (122.7429, -8.0882) (122.585, -8.0306) (122.3764, -7.9485) (122.1199, -7.8358) (121.8178, -7.6881) (121.6218, -7.5794) (121.5238, -7.5251) knots 0 0 0 0 0.033613 0.067227 0.100839 0.117647 0.134454 0.151261 0.168068 0.201677 0.210077 0.218473 0.222676 0.226878 0.231076 0.235279 0.239479 0.24368 0.247882 0.252083 0.256283 0.260485 0.268889 0.277292 0.281494 0.285694 0.289895 0.294097 0.298298 0.302498 0.306701 0.310899 0.315101 0.319304 0.3277 0.3361 0.369709 0.386516 0.403323 0.420131 0.436938 0.470551 0.504164 0.537777 0.537777 0.537777 0.537777 projected
  arc A24 (121.562, -10.0731) -> (121.6358, -10.8264) centre (141.5, -8.5) ccw projected
  spline S21 degree 3 poles (122.0928, -13.3334) (122.1784, -13.261) (122.3496, -13.1164) (122.6173, -12.9128) (122.8471, -12.7525) (123.0357, -12.6315) (123.1795, -12.5444) (123.326, -12.462) (123.5234, -12.3558) (123.7076, -12.2859) (123.852, -12.1993) (123.9069, -12.1555) (123.9467, -12.1159) (123.9731, -12.0832) (123.9972, -12.0488) (124.0177, -12.012) (124.0343, -11.9733) (124.0467, -11.9331) (124.0559, -11.892) (124.0583, -11.85) (124.0594, -11.8079) (124.0511, -11.7523) (124.0374, -11.6837) (124.026, -11.6146) (124.0141, -11.5597) (123.9983, -11.5207) (123.9812, -11.4822) (123.9581, -11.447) (123.9323, -11.4138) (123.9031, -11.3834) (123.871, -11.3562) (123.8362, -11.3325) (123.8, -11.3112) (123.7488, -11.2882) (123.682, -11.2666) (123.5163, -11.2365) (123.3193, -11.2362) (123.0971, -11.2064) (122.9309, -11.1811) (122.7657, -11.1503) (122.5465, -11.1036) (122.2749, -11.0347) (121.9526, -10.9387) (121.7414, -10.8638) (121.6358, -10.8264) knots 0 0 0 0 0.033613 0.067227 0.100839 0.117647 0.134454 0.151261 0.168068 0.201677 0.210077 0.218473 0.222676 0.226878 0.231076 0.235279 0.239479 0.24368 0.247882 0.252083 0.256283 0.260485 0.268889 0.277292 0.281494 0.285694 0.289895 0.294097 0.298298 0.302498 0.306701 0.310899 0.315101 0.319304 0.3277 0.3361 0.369709 0.386516 0.403323 0.420131 0.436938 0.470551 0.504164 0.537777 0.537777 0.537777 0.537777 projected
  arc A25 (122.0928, -13.3334) -> (122.2896, -14.0642) centre (141.5, -8.5) ccw projected
  spline S22 degree 3 poles (123.1531, -16.4617) (123.2256, -16.3763) (123.3706, -16.2055) (123.6011, -15.9606) (123.8015, -15.7647) (123.9676, -15.6143) (124.095, -15.5047) (124.226, -15.3993) (124.4032, -15.262) (124.5735, -15.1628) (124.7016, -15.0536) (124.7486, -15.0014) (124.7812, -14.9558) (124.8019, -14.9192) (124.8201, -14.8812) (124.8342, -14.8416) (124.8442, -14.8007) (124.8498, -14.759) (124.8521, -14.7169) (124.8476, -14.6751) (124.8417, -14.6334) (124.8244, -14.5799) (124.7995, -14.5145) (124.777, -14.4483) (124.7562, -14.3961) (124.7342, -14.3602) (124.711, -14.3251) (124.6824, -14.2941) (124.6515, -14.2656) (124.6177, -14.2405) (124.5815, -14.2189) (124.5434, -14.2013) (124.5041, -14.1862) (124.4498, -14.172) (124.3804, -14.1616) (124.212, -14.1592) (124.0176, -14.1913) (123.7935, -14.1985) (123.6255, -14.2009) (123.4574, -14.1977) (123.2335, -14.1877) (122.9543, -14.1645) (122.6206, -14.1229) (122.3999, -14.0837) (122.2896, -14.0642) knots 0 0 0 0 0.033613 0.067227 0.100839 0.117647 0.134454 0.151261 0.168068 0.201677 0.210077 0.218473 0.222676 0.226878 0.231076 0.235279 0.239479 0.24368 0.247882 0.252083 0.256283 0.260485 0.268889 0.277292 0.281494 0.285694 0.289895 0.294097 0.298298 0.302498 0.306701 0.310899 0.315101 0.319304 0.3277 0.3361 0.369709 0.386516 0.403323 0.420131 0.436938 0.470551 0.504164 0.537777 0.537777 0.537777 0.537777 projected
  arc A26 (123.1531, -16.4617) -> (123.4674, -17.1502) centre (141.5, -8.5) ccw projected
  spline S23 degree 3 poles (124.7137, -19.373) (124.7712, -19.2768) (124.8862, -19.0844) (125.0732, -18.8049) (125.2386, -18.5787) (125.3777, -18.403) (125.4853, -18.2739) (125.5972, -18.1484) (125.7494, -17.9839) (125.901, -17.8579) (126.0094, -17.7292) (126.0471, -17.6699) (126.0718, -17.6196) (126.0862, -17.58) (126.0979, -17.5396) (126.1053, -17.4982) (126.1084, -17.4562) (126.1071, -17.4142) (126.1024, -17.3723) (126.0911, -17.3318) (126.0784, -17.2916) (126.0525, -17.2417) (126.0173, -17.1813) (125.9841, -17.1197) (125.955, -17.0716) (125.9274, -17.0398) (125.8987, -17.009) (125.8654, -16.9832) (125.8302, -16.9601) (125.7928, -16.9409) (125.7536, -16.9256) (125.713, -16.9145) (125.6718, -16.9061) (125.616, -16.901) (125.5457, -16.9022) (125.3793, -16.9275) (125.1928, -16.9912) (124.973, -17.0352) (124.8076, -17.0652) (124.6413, -17.0897) (124.4188, -17.1167) (124.1396, -17.1398) (123.8036, -17.1536) (123.5795, -17.1513) (123.4674, -17.1502) knots 0 0 0 0 0.033613 0.067227 0.100839 0.117647 0.134454 0.151261 0.168068 0.201677 0.210077 0.218473 0.222676 0.226878 0.231076 0.235279 0.239479 0.24368 0.247882 0.252083 0.256283 0.260485 0.268889 0.277292 0.281494 0.285694 0.289895 0.294097 0.298298 0.302498 0.306701 0.310899 0.315101 0.319304 0.3277 0.3361 0.369709 0.386516 0.403323 0.420131 0.436938 0.470551 0.504164 0.537777 0.537777 0.537777 0.537777 projected
  arc A27 (124.7137, -19.373) -> (125.1371, -20.0003) centre (141.5, -8.5) ccw projected
  spline S24 degree 3 poles (126.7323, -21.9876) (126.7732, -21.8833) (126.8549, -21.6746) (126.9934, -21.3682) (127.1193, -21.1178) (127.2275, -20.9216) (127.3125, -20.7765) (127.4022, -20.6344) (127.5252, -20.447) (127.654, -20.2978) (127.7397, -20.153) (127.7672, -20.0883) (127.7833, -20.0346) (127.791, -19.9932) (127.7958, -19.9514) (127.7963, -19.9094) (127.7925, -19.8674) (127.7842, -19.8262) (127.7728, -19.7856) (127.7549, -19.7475) (127.7358, -19.71) (127.7021, -19.6651) (127.6573, -19.6113) (127.6144, -19.5559) (127.5779, -19.5133) (127.5454, -19.4865) (127.5121, -19.4608) (127.4749, -19.4408) (127.4364, -19.4239) (127.3963, -19.4111) (127.3552, -19.4025) (127.3133, -19.3982) (127.2713, -19.3967) (127.2153, -19.4008) (127.1463, -19.4136) (126.9863, -19.466) (126.8128, -19.5594) (126.6032, -19.6391) (126.4451, -19.6959) (126.2851, -19.7474) (126.0701, -19.8107) (125.7984, -19.8794) (125.4693, -19.9483) (125.2479, -19.983) (125.1371, -20.0003) knots 0 0 0 0 0.033613 0.067227 0.100839 0.117647 0.134454 0.151261 0.168068 0.201677 0.210077 0.218473 0.222676 0.226878 0.231076 0.235279 0.239479 0.24368 0.247882 0.252083 0.256283 0.260485 0.268889 0.277292 0.281494 0.285694 0.289895 0.294097 0.298298 0.302498 0.306701 0.310899 0.315101 0.319304 0.3277 0.3361 0.369709 0.386516 0.403323 0.420131 0.436938 0.470551 0.504164 0.537777 0.537777 0.537777 0.537777 projected
  arc A28 (126.7323, -21.9876) -> (127.2532, -22.5367) centre (141.5, -8.5) ccw projected